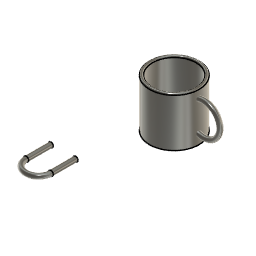
10413 안재훈 머그컵 (Autodesk Fusion 360 design; units mm, degrees)
Autodesk Fusion 360 part; units mm, degrees
sketch "스케치1" plane through (0, 0, 0) normal (0, 0, 1) x (1, 0, 0)
  circle A0 centre (0, 0) radius 50
  dimension "d1" = 100
  constraint coincident A0.centre origin
  measures "d1" diameter of A0
extrude "돌출1" add sketch "스케치1" along normal blind 100 makes body 1
shell "쉘1" thickness 6 removed faces 1 at (8.8165, -9.7599, 100) on bodies 1
fillet "필렛1" radius 3 2 edges at (-46.6164, -18.0808, 100) (-41.0224, 15.9111, 100) on bodies 1
shell "쉘2" thickness 5 removed faces 1 at (8.8165, -9.7599, 0) on bodies 1
sketch "스케치2" plane through (0, 0, 0) normal (0, 0, 1) x (1, 0, 0)
  line L0 (-50, -150) -> (-50, -200)
  arc A0 (-100, -200) -> (-50, -200) centre (-75, -200) ccw
  line L1 (-100, -200) -> (-100, -150)
  constraint vertical L0
  constraint tangent L0 A0
  constraint tangent A0 L1
  constraint parallel L0 L1
pipe "파이프1" add diameter 10 path "스케치2" along L0 A0 L1 separate body makes body 2
sketch "스케치3" plane through (0, 0, 0) normal (0, 1, 0) x (1, 0, 0)
  circle A0 centre (60, -50) radius 32.5
  dimension "d12" = 65
  measures "d12" diameter of A0
sketch "스케치4" plane through (0, 0, 0) normal (0, 1, 0) x (1, 0, 0)
pipe "파이프1'" add diameter 10 path "스케치3" along A0 separate body makes body 3 in component "Component'"
component "Component'" placed x (1, 0, 0) y (0, 1, 0) z (0, 0, 1) at (0, 0, 0)
